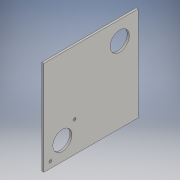
# Autodesk Inventor part: GearboxPlate
Saved by Autodesk Inventor 2016 (Build 200138000, 138)
## iProperties
Created: 2017-01-21
Part Number: GearboxPlate
Material: Generic
Document SubType Name: Modeling
Designer: Nick
Density: 1 g/cm^3
Appearance: Default
Author: Nick
Autodesk Inventor part; units mm, degrees
ref_plane "YZ Plane" through (0, 0, 0) normal (1, 0, 0) x (0, 1, 0)
ref_plane "XZ Plane" through (0, 0, 0) normal (0, 1, 0) x (-1, 0, 0)
ref_plane "XY Plane" through (0, 0, 0) normal (0, 0, 1) x (1, 0, 0)
sketch "Sketch1" plane through (0, 0, 0) normal (0, 0, 1) x (1, 0, 0)
  line L0 (-59.4683, 46.1321) -> (80.2317, 46.1321)
  line L1 (80.2317, 46.1321) -> (80.2317, -93.5679)
  line L2 (80.2317, -93.5679) -> (-59.4683, -93.5679)
  line L3 (-59.4683, -93.5679) -> (-59.4683, 46.1321)
  line L4 (-59.4683, -93.5679) -> (-5.7383, -93.5679)
  line L5 (-60.4499, -45.6669) -> (-59.4683, -93.5679)
  line L6 (-53.1183, 39.7821) -> (-11.1067, 39.7821)
  line L7 (-11.1067, 39.7821) -> (-11.1067, -2.2295)
  line L8 (-11.1067, -2.2295) -> (-53.1183, -2.2295)
  line L9 (-53.1183, -2.2295) -> (-53.1183, 39.7821)
  circle A0 centre (52.7362, -66.1162) radius 14.3002
  circle A1 centre (-32.1633, 18.7255) radius 14.1986
  circle A2 centre (-14.1547, 0.8185) radius 2.0193
  circle A3 centre (-50.0703, 36.7341) radius 2.0193
  point P0 (0, 0)
  dimension "d0" = 139.7
  dimension "d1" = 139.7
  dimension "d8" = 42.0116
  dimension "d9" = 42.0116
  dimension "d10" = 3.048
  dimension "d13" = 3.048
  dimension "d14" = 6.35
  dimension "d15" = 6.35
  dimension "d16" = 3.048
  dimension "d17" = 3.048
  dimension "d18" = 20.955
  dimension "d19" = 20.955
  dimension "d21" = 28.6004
  dimension "d23" = 120.0252
  dimension "d24" = 27.4955
  dimension "d25" = 27.4517
  dimension "d26" = 28.3972
  dimension "d27" = 4.0386
  dimension "d28" = 4.0386
  constraints: 20 end point, 4 centre point, 4 parallel, 3 coincident, 3 horizontal, 2 perpendicular
  measures "d0" distance of L0.start L0.end
  measures "d1" distance of L0.end L1.end
  measures "d8" distance of L6.end L7.end
  measures "d9" distance of L7.end L8.end
  measures "d10" distance from line of L6 point (-50.07, 36.734)
  measures "d13" distance from line of L8 point (-14.155, 0.818)
  measures "d14" distance between parallel lines of L6 L0
  measures "d15" distance between parallel lines of L3 L9
  measures "d16" distance from line of L7 point (-14.155, 0.818)
  measures "d17" distance from line of L9 point (-50.07, 36.734)
  measures "d18" distance from line of L8 point (-32.163, 18.725)
  measures "d19" distance from line of L9 point (-32.163, 18.725)
  measures "d21" diameter of A0
  measures "d23" distance of A0.centre point (-32.163, 18.725)
  measures "d24" distance from line of L1 A0.centre
  measures "d25" distance from line of L2 A0.centre
  measures "d26" diameter of A1
  measures "d27" diameter of A3
  measures "d28" diameter of A2
extrude "Extrusion1" add sketch "Sketch1" along normal blind 3.175 contours L0 L1 L2 L3 | L6 L7 L8 L9
body "Solid1"
